Autodesk Inventor part; units mm, degrees
(part 3 of 3)
sketch "Эскиз4" plane through (0, 0, 0) normal (0, 0, -1) x (-1, 0, 0)
  arc A0 (-8.5879, 10.673) -> (-10.7903, 9.2375) centre (-9.1909, 9.1909) ccw
  line L0 (-8.8865, 7.6202) -> (-10.7903, 9.2375)
  arc A1 (-8.8865, 7.6202) -> (-7.8258, 10.0255) centre (-9.1909, 9.1909) ccw
  line L1 (-7.2868, 10.66) -> (-7.8258, 10.0255)
  line L2 (-8.5879, 10.673) -> (-8.0489, 11.3074)
  line L3 (-8.185, 11.3816) -> (-8.0489, 11.3074)
  line L4 (-8.4933, 11.4983) -> (-8.185, 11.3816)
  line L5 (-9.1961, 12.0463) -> (-8.4933, 11.4983)
  line L6 (-9.9839, 14.2526) -> (-9.1961, 12.0463)
  line L7 (-9.6596, 14.7646) -> (-9.9839, 14.2526)
  line L8 (-9.2928, 14.7834) -> (-9.6596, 14.7646)
  line L9 (-8.9255, 14.778) -> (-9.2928, 14.7834)
  line L10 (-8.5594, 14.7485) -> (-8.9255, 14.778)
  line L11 (-8.196, 14.6951) -> (-8.5594, 14.7485)
  line L12 (-7.837, 14.618) -> (-8.196, 14.6951)
  line L13 (-7.4837, 14.5174) -> (-7.837, 14.618)
  line L14 (-7.1378, 14.3939) -> (-7.4837, 14.5174)
  line L15 (-6.8007, 14.2479) -> (-7.1378, 14.3939)
  line L16 (-6.474, 14.0801) -> (-6.8007, 14.2479)
  line L17 (-6.159, 13.8913) -> (-6.474, 14.0801)
  line L18 (-5.857, 13.6822) -> (-6.159, 13.8913)
  line L19 (-5.5695, 13.4537) -> (-5.857, 13.6822)
  line L20 (-5.2975, 13.2068) -> (-5.5695, 13.4537)
  line L21 (-5.0423, 12.9426) -> (-5.2975, 13.2068)
  line L22 (-4.8051, 12.6623) -> (-5.0423, 12.9426)
  line L23 (-4.5867, 12.3669) -> (-4.8051, 12.6623)
  line L24 (-4.3882, 12.0579) -> (-4.5867, 12.3669)
  line L25 (-4.2104, 11.7365) -> (-4.3882, 12.0579)
  line L26 (-4.0541, 11.4041) -> (-4.2104, 11.7365)
  line L27 (-3.9199, 11.0622) -> (-4.0541, 11.4041)
  line L28 (-3.8084, 10.7123) -> (-3.9199, 11.0622)
  line L29 (-3.7202, 10.3557) -> (-3.8084, 10.7123)
  line L30 (-3.6555, 9.9942) -> (-3.7202, 10.3557)
  line L31 (-3.6147, 9.6291) -> (-3.6555, 9.9942)
  line L32 (-4.0677, 9.2263) -> (-3.6147, 9.6291)
  line L33 (-6.3723, 9.6472) -> (-4.0677, 9.2263)
  line L34 (-7.0266, 10.2523) -> (-6.3723, 9.6472)
  line L35 (-7.1917, 10.5377) -> (-7.0266, 10.2523)
  line L36 (-7.2868, 10.66) -> (-7.1917, 10.5377)
  line L37 (-7.2868, 10.66) -> (-7.8258, 10.0255)
  arc A2 (-8.8865, 7.6202) -> (-7.8258, 10.0255) centre (-9.1909, 9.1909) ccw
  line L38 (-8.8865, 7.6202) -> (-10.7903, 9.2375)
  arc A3 (-8.5879, 10.673) -> (-10.7903, 9.2375) centre (-9.1909, 9.1909) ccw
  line L39 (-8.5848, 2.046) -> (-8.6119, 2.08)
  line L40 (-8.5619, 2.0118) -> (-8.5848, 2.046)
  line L41 (-8.5252, 1.9426) -> (-8.5619, 2.0118)
  line L42 (-8.4969, 1.8728) -> (-8.5252, 1.9426)
  line L43 (-8.4749, 1.8024) -> (-8.4969, 1.8728)
  line L44 (-8.4578, 1.7316) -> (-8.4749, 1.8024)
  line L45 (-8.4351, 1.5888) -> (-8.4578, 1.7316)
  line L46 (-8.3988, 1.4474) -> (-8.4351, 1.5888)
  line L47 (-8.348, 1.3076) -> (-8.3988, 1.4474)
  line L48 (-8.2864, 1.1692) -> (-8.348, 1.3076)
  line L49 (-8.2156, 1.0322) -> (-8.2864, 1.1692)
  line L50 (-8.1367, 0.8965) -> (-8.2156, 1.0322)
  line L51 (-8.0501, 0.7623) -> (-8.1367, 0.8965)
  line L52 (-7.9562, 0.6297) -> (-8.0501, 0.7623)
  line L53 (-7.8555, 0.4989) -> (-7.9562, 0.6297)
  line L54 (-7.7481, 0.3698) -> (-7.8555, 0.4989)
  line L55 (-7.6343, 0.2426) -> (-7.7481, 0.3698)
  line L56 (-7.5448, 0.1486) -> (-7.6343, 0.2426)
  line L57 (-6.9702, 0.2723) -> (-7.5448, 0.1486)
  line L58 (-6.9273, 0.3948) -> (-6.9702, 0.2723)
  line L59 (-6.8759, 0.5575) -> (-6.9273, 0.3948)
  line L60 (-6.8312, 0.7194) -> (-6.8759, 0.5575)
  line L61 (-6.7932, 0.8801) -> (-6.8312, 0.7194)
  line L62 (-6.7622, 1.0396) -> (-6.7932, 0.8801)
  line L63 (-6.7385, 1.1975) -> (-6.7622, 1.0396)
  line L64 (-6.7224, 1.3537) -> (-6.7385, 1.1975)
  line L65 (-6.7143, 1.5077) -> (-6.7224, 1.3537)
  line L66 (-6.7151, 1.6592) -> (-6.7143, 1.5077)
  line L67 (-6.7263, 1.8075) -> (-6.7151, 1.6592)
  line L68 (-6.7515, 1.9513) -> (-6.7263, 1.8075)
  line L69 (-6.7895, 2.0908) -> (-6.7515, 1.9513)
  line L70 (-6.8031, 2.1623) -> (-6.7895, 2.0908)
  line L71 (-6.812, 2.2355) -> (-6.8031, 2.1623)
  line L72 (-6.8149, 2.3108) -> (-6.812, 2.2355)
  line L73 (-6.8099, 2.389) -> (-6.8149, 2.3108)
  line L74 (-6.8032, 2.4296) -> (-6.8099, 2.389)
  line L75 (-6.7924, 2.4717) -> (-6.8032, 2.4296)
  line L76 (-6.7757, 2.516) -> (-6.7924, 2.4717)
  line L77 (-6.7479, 2.5646) -> (-6.7757, 2.516)
  line L78 (-6.6571, 2.6374) -> (-6.7479, 2.5646)
  line L79 (-6.1482, 2.8577) -> (-6.6571, 2.6374)
  line L80 (-6.0329, 2.874) -> (-6.1482, 2.8577)
  line L81 (-5.9785, 2.861) -> (-6.0329, 2.874)
  line L82 (-5.9347, 2.8428) -> (-5.9785, 2.861)
  line L83 (-5.8967, 2.8219) -> (-5.9347, 2.8428)
  line L84 (-5.8625, 2.799) -> (-5.8967, 2.8219)
  line L85 (-5.8021, 2.7491) -> (-5.8625, 2.799)
  line L86 (-5.7492, 2.6954) -> (-5.8021, 2.7491)
  line L87 (-5.7019, 2.6389) -> (-5.7492, 2.6954)
  line L88 (-5.6591, 2.5799) -> (-5.7019, 2.6389)
  line L89 (-5.5834, 2.4568) -> (-5.6591, 2.5799)
  line L90 (-5.4958, 2.34) -> (-5.5834, 2.4568)
  line L91 (-5.3953, 2.2303) -> (-5.4958, 2.34)
  line L92 (-5.2855, 2.126) -> (-5.3953, 2.2303)
  line L93 (-5.1677, 2.0265) -> (-5.2855, 2.126)
  line L94 (-5.0428, 1.9313) -> (-5.1677, 2.0265)
  line L95 (-4.9114, 1.8405) -> (-5.0428, 1.9313)
  line L96 (-4.774, 1.7539) -> (-4.9114, 1.8405)
  line L97 (-4.6308, 1.6716) -> (-4.774, 1.7539)
  line L98 (-4.4822, 1.5934) -> (-4.6308, 1.6716)
  line L99 (-4.3284, 1.5195) -> (-4.4822, 1.5934)
  line L100 (-4.2097, 1.4669) -> (-4.3284, 1.5195)
  line L101 (-3.7262, 1.8011) -> (-4.2097, 1.4669)
  line L102 (-3.7335, 1.9306) -> (-3.7262, 1.8011)
  line L103 (-3.7483, 2.1006) -> (-3.7335, 1.9306)
  line L104 (-3.7689, 2.2673) -> (-3.7483, 2.1006)
  line L105 (-3.7953, 2.4303) -> (-3.7689, 2.2673)
  line L106 (-3.8277, 2.5895) -> (-3.7953, 2.4303)
  line L107 (-3.8662, 2.7445) -> (-3.8277, 2.5895)
  line L108 (-3.9111, 2.8949) -> (-3.8662, 2.7445)
  line L109 (-3.9626, 3.0403) -> (-3.9111, 2.8949)
  line L110 (-4.0213, 3.18) -> (-3.9626, 3.0403)
  line L111 (-4.0884, 3.3127) -> (-4.0213, 3.18)
  line L112 (-4.1667, 3.4359) -> (-4.0884, 3.3127)
  line L113 (-4.2551, 3.5502) -> (-4.1667, 3.4359)
  line L114 (-4.2951, 3.6112) -> (-4.2551, 3.5502)
  line L115 (-4.3313, 3.6754) -> (-4.2951, 3.6112)
  line L116 (-4.3629, 3.7438) -> (-4.3313, 3.6754)
  line L117 (-4.3881, 3.8179) -> (-4.3629, 3.7438)
  line L118 (-4.3975, 3.858) -> (-4.3881, 3.8179)
  line L119 (-4.4036, 3.901) -> (-4.3975, 3.858)
  line L120 (-4.4051, 3.9484) -> (-4.4036, 3.901)
  line L121 (-4.398, 4.0039) -> (-4.4051, 3.9484)
  line L122 (-4.3421, 4.106) -> (-4.398, 4.0039)
  line L123 (-3.9562, 4.5042) -> (-4.3421, 4.106)
  line L124 (-3.8559, 4.5633) -> (-3.9562, 4.5042)
  line L125 (-3.8007, 4.5722) -> (-3.8559, 4.5633)
  line L126 (-3.7533, 4.5722) -> (-3.8007, 4.5722)
  line L127 (-3.7101, 4.5673) -> (-3.7533, 4.5722)
  line L128 (-3.6697, 4.5593) -> (-3.7101, 4.5673)
  line L129 (-3.5949, 4.5364) -> (-3.6697, 4.5593)
  line L130 (-3.5255, 4.507) -> (-3.5949, 4.5364)
  line L131 (-3.4601, 4.4728) -> (-3.5255, 4.507)
  line L132 (-3.398, 4.4348) -> (-3.4601, 4.4728)
  line L133 (-3.2809, 4.3499) -> (-3.398, 4.4348)
  line L134 (-3.1554, 4.2755) -> (-3.2809, 4.3499)
  line L135 (-3.0205, 4.2127) -> (-3.1554, 4.2755)
  line L136 (-2.8791, 4.1584) -> (-3.0205, 4.2127)
  line L137 (-2.7322, 4.1115) -> (-2.8791, 4.1584)
  line L138 (-2.5804, 4.0714) -> (-2.7322, 4.1115)
  line L139 (-2.4243, 4.0377) -> (-2.5804, 4.0714)
  line L140 (-2.2642, 4.0103) -> (-2.4243, 4.0377)
  line L141 (-2.1004, 3.989) -> (-2.2642, 4.0103)
  line L142 (-1.9332, 3.9737) -> (-2.1004, 3.989)
  line L143 (-1.7628, 3.9643) -> (-1.9332, 3.9737)
  line L144 (-1.6331, 3.961) -> (-1.7628, 3.9643)
  line L145 (-1.3142, 4.4548) -> (-1.6331, 3.961)
  line L146 (-1.3705, 4.5717) -> (-1.3142, 4.4548)
  line L147 (-1.4492, 4.7232) -> (-1.3705, 4.5717)
  line L148 (-1.532, 4.8692) -> (-1.4492, 4.7232)
  line L149 (-1.6189, 5.0098) -> (-1.532, 4.8692)
  line L150 (-1.7097, 5.1444) -> (-1.6189, 5.0098)
  line L151 (-1.8046, 5.2729) -> (-1.7097, 5.1444)
  line L152 (-1.9036, 5.3947) -> (-1.8046, 5.2729)
  line L153 (-2.0068, 5.5093) -> (-1.9036, 5.3947)
  line L154 (-2.1145, 5.6158) -> (-2.0068, 5.5093)
  line L155 (-2.2273, 5.7129) -> (-2.1145, 5.6158)
  line L156 (-2.3468, 5.7967) -> (-2.2273, 5.7129)
  line L157 (-2.4723, 5.8685) -> (-2.3468, 5.7967)
  line L158 (-2.5325, 5.9094) -> (-2.4723, 5.8685)
  line L159 (-2.5905, 5.9549) -> (-2.5325, 5.9094)
  line L160 (-2.6459, 6.0061) -> (-2.5905, 5.9549)
  line L161 (-2.6976, 6.0649) -> (-2.6459, 6.0061)
  line L162 (-2.7215, 6.0983) -> (-2.6976, 6.0649)
  line L163 (-2.7437, 6.1357) -> (-2.7215, 6.0983)
  line L164 (-2.7632, 6.1789) -> (-2.7437, 6.1357)
  line L165 (-2.7779, 6.2329) -> (-2.7632, 6.1789)
  line L166 (-2.7652, 6.3486) -> (-2.7779, 6.2329)
  line L167 (-2.5611, 6.8642) -> (-2.7652, 6.3486)
  line L168 (-2.4911, 6.9572) -> (-2.5611, 6.8642)
  line L169 (-2.4434, 6.9865) -> (-2.4911, 6.9572)
  line L170 (-2.3996, 7.0047) -> (-2.4434, 6.9865)
  line L171 (-2.3579, 7.0167) -> (-2.3996, 7.0047)
  line L172 (-2.3175, 7.0247) -> (-2.3579, 7.0167)
  line L173 (-2.2396, 7.0322) -> (-2.3175, 7.0247)
  line L174 (-2.1643, 7.0316) -> (-2.2396, 7.0322)
  line L175 (-2.0908, 7.025) -> (-2.1643, 7.0316)
  line L176 (-2.0188, 7.0137) -> (-2.0908, 7.025)
  line L177 (-1.8782, 6.9801) -> (-2.0188, 7.0137)
  line L178 (-1.7338, 6.9594) -> (-1.8782, 6.9801)
  line L179 (-1.5851, 6.9529) -> (-1.7338, 6.9594)
  line L180 (-1.4337, 6.9569) -> (-1.5851, 6.9529)
  line L181 (-1.28, 6.9698) -> (-1.4337, 6.9569)
  line L182 (-1.1244, 6.9908) -> (-1.28, 6.9698)
  line L183 (-0.9673, 7.0195) -> (-1.1244, 6.9908)
  line L184 (-0.8089, 7.0554) -> (-0.9673, 7.0195)
  line L185 (-0.6494, 7.0984) -> (-0.8089, 7.0554)
  line L186 (-0.4891, 7.1482) -> (-0.6494, 7.0984)
  line L187 (-0.3281, 7.2047) -> (-0.4891, 7.1482)
  line L188 (-0.207, 7.2514) -> (-0.3281, 7.2047)
  line L189 (-0.1014, 7.8296) -> (-0.207, 7.2514)
  line L190 (-0.1981, 7.9161) -> (-0.1014, 7.8296)
  line L191 (-0.3288, 8.0259) -> (-0.1981, 7.9161)
  line L192 (-0.4612, 8.1291) -> (-0.3288, 8.0259)
  line L193 (-0.5952, 8.2257) -> (-0.4612, 8.1291)
  line L194 (-0.7307, 8.3154) -> (-0.5952, 8.2257)
  line L195 (-0.8675, 8.3977) -> (-0.7307, 8.3154)
  line L196 (-1.0056, 8.4724) -> (-0.8675, 8.3977)
  line L197 (-1.1448, 8.5388) -> (-1.0056, 8.4724)
  line L198 (-1.2851, 8.596) -> (-1.1448, 8.5388)
  line L199 (-1.4264, 8.6425) -> (-1.2851, 8.596)
  line L200 (-1.5688, 8.6742) -> (-1.4264, 8.6425)
  line L201 (-1.7122, 8.6925) -> (-1.5688, 8.6742)
  line L202 (-1.7836, 8.7073) -> (-1.7122, 8.6925)
  line L203 (-1.8546, 8.7271) -> (-1.7836, 8.7073)
  line L204 (-1.9253, 8.7532) -> (-1.8546, 8.7271)
  line L205 (-1.9955, 8.7878) -> (-1.9253, 8.7532)
  line L206 (-2.0305, 8.8095) -> (-1.9955, 8.7878)
  line L207 (-2.0653, 8.8355) -> (-2.0305, 8.8095)
  line L208 (-2.0998, 8.868) -> (-2.0653, 8.8355)
  line L209 (-2.1341, 8.9122) -> (-2.0998, 8.868)
  line L210 (-2.1666, 9.024) -> (-2.1341, 8.9122)
  line L211 (-2.1753, 9.5784) -> (-2.1666, 9.024)
  line L212 (-2.1463, 9.6911) -> (-2.1753, 9.5784)
  line L213 (-2.1135, 9.7365) -> (-2.1463, 9.6911)
  line L214 (-2.08, 9.77) -> (-2.1135, 9.7365)
  line L215 (-2.046, 9.7971) -> (-2.08, 9.77)
  line L216 (-2.0118, 9.8199) -> (-2.046, 9.7971)
  line L217 (-1.9426, 9.8567) -> (-2.0118, 9.8199)
  line L218 (-1.8728, 9.885) -> (-1.9426, 9.8567)
  line L219 (-1.8024, 9.907) -> (-1.8728, 9.885)
  line L220 (-1.7316, 9.924) -> (-1.8024, 9.907)
  line L221 (-1.5888, 9.9468) -> (-1.7316, 9.924)
  line L222 (-1.4474, 9.983) -> (-1.5888, 9.9468)
  line L223 (-1.3076, 10.0339) -> (-1.4474, 9.983)
  line L224 (-1.1692, 10.0955) -> (-1.3076, 10.0339)
  line L225 (-1.0322, 10.1662) -> (-1.1692, 10.0955)
  line L226 (-0.8965, 10.2452) -> (-1.0322, 10.1662)
  line L227 (-0.7623, 10.3318) -> (-0.8965, 10.2452)
  line L228 (-0.6297, 10.4256) -> (-0.7623, 10.3318)
  line L229 (-0.4989, 10.5264) -> (-0.6297, 10.4256)
  line L230 (-0.3698, 10.6338) -> (-0.4989, 10.5264)
  line L231 (-0.2426, 10.7476) -> (-0.3698, 10.6338)
  line L232 (-0.1486, 10.8371) -> (-0.2426, 10.7476)
  line L233 (-0.2723, 11.4117) -> (-0.1486, 10.8371)
  line L234 (-0.3948, 11.4545) -> (-0.2723, 11.4117)
  line L235 (-0.5575, 11.506) -> (-0.3948, 11.4545)
  line L236 (-0.7194, 11.5507) -> (-0.5575, 11.506)
  line L237 (-0.8801, 11.5887) -> (-0.7194, 11.5507)
  line L238 (-1.0396, 11.6196) -> (-0.8801, 11.5887)
  line L239 (-1.1975, 11.6434) -> (-1.0396, 11.6196)
  line L240 (-1.3537, 11.6595) -> (-1.1975, 11.6434)
  line L241 (-1.5077, 11.6676) -> (-1.3537, 11.6595)
  line L242 (-1.6592, 11.6667) -> (-1.5077, 11.6676)
  line L243 (-1.8075, 11.6556) -> (-1.6592, 11.6667)
  line L244 (-1.9513, 11.6304) -> (-1.8075, 11.6556)
  line L245 (-2.0908, 11.5924) -> (-1.9513, 11.6304)
  line L246 (-2.1623, 11.5788) -> (-2.0908, 11.5924)
  line L247 (-2.2355, 11.5699) -> (-2.1623, 11.5788)
  line L248 (-2.3108, 11.567) -> (-2.2355, 11.5699)
  line L249 (-2.389, 11.572) -> (-2.3108, 11.567)
  line L250 (-2.4296, 11.5787) -> (-2.389, 11.572)
  line L251 (-2.4717, 11.5894) -> (-2.4296, 11.5787)
  line L252 (-2.516, 11.6062) -> (-2.4717, 11.5894)
  line L253 (-2.5646, 11.634) -> (-2.516, 11.6062)
  line L254 (-2.6374, 11.7248) -> (-2.5646, 11.634)
  line L255 (-2.8577, 12.2337) -> (-2.6374, 11.7248)
  line L256 (-2.874, 12.3489) -> (-2.8577, 12.2337)
  line L257 (-2.861, 12.4034) -> (-2.874, 12.3489)
  line L258 (-2.8428, 12.4472) -> (-2.861, 12.4034)
  line L259 (-2.8219, 12.4852) -> (-2.8428, 12.4472)
  line L260 (-2.799, 12.5194) -> (-2.8219, 12.4852)
  line L261 (-2.7491, 12.5798) -> (-2.799, 12.5194)
  line L262 (-2.6954, 12.6327) -> (-2.7491, 12.5798)
  line L263 (-2.6389, 12.6799) -> (-2.6954, 12.6327)
  line L264 (-2.5799, 12.7228) -> (-2.6389, 12.6799)
  line L265 (-2.4568, 12.7985) -> (-2.5799, 12.7228)
  line L266 (-2.34, 12.886) -> (-2.4568, 12.7985)
  line L267 (-2.2303, 12.9865) -> (-2.34, 12.886)
  line L268 (-2.126, 13.0964) -> (-2.2303, 12.9865)
  line L269 (-2.0265, 13.2142) -> (-2.126, 13.0964)
  line L270 (-1.9313, 13.3391) -> (-2.0265, 13.2142)
  line L271 (-1.8405, 13.4704) -> (-1.9313, 13.3391)
  line L272 (-1.7539, 13.6079) -> (-1.8405, 13.4704)
  line L273 (-1.6716, 13.7511) -> (-1.7539, 13.6079)
  line L274 (-1.5934, 13.8997) -> (-1.6716, 13.7511)
  line L275 (-1.5195, 14.0535) -> (-1.5934, 13.8997)
  line L276 (-1.4669, 14.1721) -> (-1.5195, 14.0535)
  line L277 (-1.8011, 14.6556) -> (-1.4669, 14.1721)
  line L278 (-1.9306, 14.6484) -> (-1.8011, 14.6556)
  line L279 (-2.1006, 14.6336) -> (-1.9306, 14.6484)
  line L280 (-2.2673, 14.613) -> (-2.1006, 14.6336)
  line L281 (-2.4303, 14.5866) -> (-2.2673, 14.613)
  line L282 (-2.5895, 14.5541) -> (-2.4303, 14.5866)
  line L283 (-2.7445, 14.5156) -> (-2.5895, 14.5541)
  line L284 (-2.8949, 14.4708) -> (-2.7445, 14.5156)
  line L285 (-3.0403, 14.4193) -> (-2.8949, 14.4708)
  line L286 (-3.18, 14.3605) -> (-3.0403, 14.4193)
  line L287 (-3.3127, 14.2935) -> (-3.18, 14.3605)
  line L288 (-3.4359, 14.2152) -> (-3.3127, 14.2935)
  line L289 (-3.5502, 14.1267) -> (-3.4359, 14.2152)
  line L290 (-3.6112, 14.0868) -> (-3.5502, 14.1267)
  line L291 (-3.6754, 14.0505) -> (-3.6112, 14.0868)
  line L292 (-3.7438, 14.019) -> (-3.6754, 14.0505)
  line L293 (-3.8179, 13.9938) -> (-3.7438, 14.019)
  line L294 (-3.858, 13.9844) -> (-3.8179, 13.9938)
  line L295 (-3.901, 13.9782) -> (-3.858, 13.9844)
  line L296 (-3.9484, 13.9767) -> (-3.901, 13.9782)
  line L297 (-4.0039, 13.9838) -> (-3.9484, 13.9767)
  line L298 (-4.106, 14.0398) -> (-4.0039, 13.9838)
  line L299 (-4.5042, 14.4257) -> (-4.106, 14.0398)
  line L300 (-4.5633, 14.5259) -> (-4.5042, 14.4257)
  line L301 (-4.5722, 14.5812) -> (-4.5633, 14.5259)
  line L302 (-4.5722, 14.6286) -> (-4.5722, 14.5812)
  line L303 (-4.5673, 14.6718) -> (-4.5722, 14.6286)
  line L304 (-4.5593, 14.7121) -> (-4.5673, 14.6718)
  line L305 (-4.5364, 14.787) -> (-4.5593, 14.7121)
  line L306 (-4.507, 14.8564) -> (-4.5364, 14.787)
  line L307 (-4.4728, 14.9217) -> (-4.507, 14.8564)
  line L308 (-4.4348, 14.9839) -> (-4.4728, 14.9217)
  line L309 (-4.3499, 15.1009) -> (-4.4348, 14.9839)
  line L310 (-4.2755, 15.2265) -> (-4.3499, 15.1009)
  line L311 (-4.2127, 15.3613) -> (-4.2755, 15.2265)
  line L312 (-4.1584, 15.5028) -> (-4.2127, 15.3613)
  line L313 (-4.1115, 15.6497) -> (-4.1584, 15.5028)
  line L314 (-4.0714, 15.8015) -> (-4.1115, 15.6497)
  line L315 (-4.0377, 15.9576) -> (-4.0714, 15.8015)
  line L316 (-4.0103, 16.1177) -> (-4.0377, 15.9576)
  line L317 (-3.989, 16.2815) -> (-4.0103, 16.1177)
  line L318 (-3.9737, 16.4487) -> (-3.989, 16.2815)
  line L319 (-3.9643, 16.6191) -> (-3.9737, 16.4487)
  line L320 (-3.961, 16.7488) -> (-3.9643, 16.6191)
  line L321 (-4.4548, 17.0676) -> (-3.961, 16.7488)
  line L322 (-4.5717, 17.0113) -> (-4.4548, 17.0676)
  line L323 (-4.7232, 16.9326) -> (-4.5717, 17.0113)
  line L324 (-4.8692, 16.8498) -> (-4.7232, 16.9326)
  line L325 (-5.0098, 16.763) -> (-4.8692, 16.8498)
  line L326 (-5.1444, 16.6721) -> (-5.0098, 16.763)
  line L327 (-5.2729, 16.5772) -> (-5.1444, 16.6721)
  line L328 (-5.3947, 16.4783) -> (-5.2729, 16.5772)
  line L329 (-5.5093, 16.375) -> (-5.3947, 16.4783)
  line L330 (-5.6158, 16.2673) -> (-5.5093, 16.375)
  line L331 (-5.7129, 16.1546) -> (-5.6158, 16.2673)
  line L332 (-5.7967, 16.0351) -> (-5.7129, 16.1546)
  line L333 (-5.8685, 15.9096) -> (-5.7967, 16.0351)
  line L334 (-5.9094, 15.8494) -> (-5.8685, 15.9096)
  line L335 (-5.9549, 15.7913) -> (-5.9094, 15.8494)
  line L336 (-6.0061, 15.736) -> (-5.9549, 15.7913)
  line L337 (-6.0649, 15.6843) -> (-6.0061, 15.736)
  line L338 (-6.0983, 15.6603) -> (-6.0649, 15.6843)
  line L339 (-6.1357, 15.6382) -> (-6.0983, 15.6603)
  line L340 (-6.1789, 15.6187) -> (-6.1357, 15.6382)
  line L341 (-6.2329, 15.604) -> (-6.1789, 15.6187)
  line L342 (-6.3486, 15.6166) -> (-6.2329, 15.604)
  line L343 (-6.8642, 15.8208) -> (-6.3486, 15.6166)
  line L344 (-6.9572, 15.8907) -> (-6.8642, 15.8208)
  line L345 (-6.9865, 15.9384) -> (-6.9572, 15.8907)
  line L346 (-7.0047, 15.9822) -> (-6.9865, 15.9384)
  line L347 (-7.0167, 16.0239) -> (-7.0047, 15.9822)
  line L348 (-7.0247, 16.0643) -> (-7.0167, 16.0239)
  line L349 (-7.0322, 16.1423) -> (-7.0247, 16.0643)
  line L350 (-7.0316, 16.2176) -> (-7.0322, 16.1423)
  line L351 (-7.025, 16.2911) -> (-7.0316, 16.2176)
  line L352 (-7.0137, 16.363) -> (-7.025, 16.2911)
  line L353 (-6.9801, 16.5036) -> (-7.0137, 16.363)
  line L354 (-6.9594, 16.6481) -> (-6.9801, 16.5036)
  line L355 (-6.9529, 16.7967) -> (-6.9594, 16.6481)
  line L356 (-6.9569, 16.9482) -> (-6.9529, 16.7967)
  line L357 (-6.9698, 17.1019) -> (-6.9569, 16.9482)
  line L358 (-6.9908, 17.2574) -> (-6.9698, 17.1019)
  line L359 (-7.0195, 17.4145) -> (-6.9908, 17.2574)
  line L360 (-7.0554, 17.5729) -> (-7.0195, 17.4145)
  line L361 (-7.0984, 17.7324) -> (-7.0554, 17.5729)
  line L362 (-7.1482, 17.8928) -> (-7.0984, 17.7324)
  line L363 (-7.2047, 18.0538) -> (-7.1482, 17.8928)
  line L364 (-7.2514, 18.1749) -> (-7.2047, 18.0538)
  line L365 (-7.8296, 18.2805) -> (-7.2514, 18.1749)
  line L366 (-7.9161, 18.1837) -> (-7.8296, 18.2805)
  line L367 (-8.0259, 18.0531) -> (-7.9161, 18.1837)
  line L368 (-8.1291, 17.9207) -> (-8.0259, 18.0531)
  line L369 (-8.2257, 17.7867) -> (-8.1291, 17.9207)
  line L370 (-8.3154, 17.6512) -> (-8.2257, 17.7867)
  line L371 (-8.3977, 17.5144) -> (-8.3154, 17.6512)
  line L372 (-8.4724, 17.3763) -> (-8.3977, 17.5144)
  line L373 (-8.5388, 17.2371) -> (-8.4724, 17.3763)
  line L374 (-8.596, 17.0968) -> (-8.5388, 17.2371)
  line L375 (-8.6425, 16.9555) -> (-8.596, 17.0968)
  line L376 (-8.6742, 16.813) -> (-8.6425, 16.9555)
  line L377 (-8.6925, 16.6696) -> (-8.6742, 16.813)
  line L378 (-8.7073, 16.5983) -> (-8.6925, 16.6696)
  line L379 (-8.7271, 16.5273) -> (-8.7073, 16.5983)
  line L380 (-8.7532, 16.4566) -> (-8.7271, 16.5273)
  line L381 (-8.7878, 16.3863) -> (-8.7532, 16.4566)
  line L382 (-8.8095, 16.3514) -> (-8.7878, 16.3863)
  line L383 (-8.8355, 16.3166) -> (-8.8095, 16.3514)
  line L384 (-8.868, 16.282) -> (-8.8355, 16.3166)
  line L385 (-8.9122, 16.2478) -> (-8.868, 16.282)
  line L386 (-9.024, 16.2152) -> (-8.9122, 16.2478)
  line L387 (-9.5784, 16.2065) -> (-9.024, 16.2152)
  line L388 (-9.6911, 16.2356) -> (-9.5784, 16.2065)
  line L389 (-9.7365, 16.2684) -> (-9.6911, 16.2356)
  line L390 (-9.77, 16.3019) -> (-9.7365, 16.2684)
  line L391 (-9.7971, 16.3359) -> (-9.77, 16.3019)
  line L392 (-9.8199, 16.3701) -> (-9.7971, 16.3359)
  line L393 (-9.8567, 16.4393) -> (-9.8199, 16.3701)
  line L394 (-9.885, 16.5091) -> (-9.8567, 16.4393)
  line L395 (-9.907, 16.5795) -> (-9.885, 16.5091)
  line L396 (-9.924, 16.6503) -> (-9.907, 16.5795)
  line L397 (-9.9468, 16.7931) -> (-9.924, 16.6503)
  line L398 (-9.983, 16.9344) -> (-9.9468, 16.7931)
  line L399 (-10.0339, 17.0742) -> (-9.983, 16.9344)
  line L400 (-10.0955, 17.2126) -> (-10.0339, 17.0742)
  line L401 (-10.1662, 17.3497) -> (-10.0955, 17.2126)
  line L402 (-10.2452, 17.4854) -> (-10.1662, 17.3497)
  line L403 (-10.3318, 17.6195) -> (-10.2452, 17.4854)
  line L404 (-10.4256, 17.7521) -> (-10.3318, 17.6195)
  line L405 (-10.5264, 17.883) -> (-10.4256, 17.7521)
  line L406 (-10.6338, 18.0121) -> (-10.5264, 17.883)
  line L407 (-10.7476, 18.1392) -> (-10.6338, 18.0121)
  line L408 (-10.8371, 18.2332) -> (-10.7476, 18.1392)
  line L409 (-11.4117, 18.1095) -> (-10.8371, 18.2332)
  line L410 (-11.4545, 17.987) -> (-11.4117, 18.1095)
  line L411 (-11.506, 17.8243) -> (-11.4545, 17.987)
  line L412 (-11.5507, 17.6625) -> (-11.506, 17.8243)
  line L413 (-11.5887, 17.5017) -> (-11.5507, 17.6625)
  line L414 (-11.6196, 17.3423) -> (-11.5887, 17.5017)
  line L415 (-11.6434, 17.1843) -> (-11.6196, 17.3423)
  line L416 (-11.6595, 17.0282) -> (-11.6434, 17.1843)
  line L417 (-11.6676, 16.8742) -> (-11.6595, 17.0282)
  line L418 (-11.6667, 16.7227) -> (-11.6676, 16.8742)
  line L419 (-11.6556, 16.5743) -> (-11.6667, 16.7227)
  line L420 (-11.6304, 16.4306) -> (-11.6556, 16.5743)
  line L421 (-11.5924, 16.2911) -> (-11.6304, 16.4306)
  line L422 (-11.5788, 16.2195) -> (-11.5924, 16.2911)
  line L423 (-11.5699, 16.1463) -> (-11.5788, 16.2195)
  line L424 (-11.567, 16.071) -> (-11.5699, 16.1463)
  line L425 (-11.572, 15.9929) -> (-11.567, 16.071)
  line L426 (-11.5787, 15.9523) -> (-11.572, 15.9929)
  line L427 (-11.5894, 15.9102) -> (-11.5787, 15.9523)
  line L428 (-11.6062, 15.8658) -> (-11.5894, 15.9102)
  line L429 (-11.634, 15.8173) -> (-11.6062, 15.8658)
  line L430 (-11.7248, 15.7444) -> (-11.634, 15.8173)
  line L431 (-12.2337, 15.5242) -> (-11.7248, 15.7444)
  line L432 (-12.3489, 15.5079) -> (-12.2337, 15.5242)
  line L433 (-12.4034, 15.5209) -> (-12.3489, 15.5079)
  line L434 (-12.4472, 15.539) -> (-12.4034, 15.5209)
  line L435 (-12.4852, 15.56) -> (-12.4472, 15.539)
  line L436 (-12.5194, 15.5829) -> (-12.4852, 15.56)
  line L437 (-12.5798, 15.6327) -> (-12.5194, 15.5829)
  line L438 (-12.6327, 15.6864) -> (-12.5798, 15.6327)
  line L439 (-12.6799, 15.743) -> (-12.6327, 15.6864)
  line L440 (-12.7228, 15.8019) -> (-12.6799, 15.743)
  line L441 (-12.7985, 15.9251) -> (-12.7228, 15.8019)
  line L442 (-12.886, 16.0419) -> (-12.7985, 15.9251)
  line L443 (-12.9865, 16.1515) -> (-12.886, 16.0419)
  line L444 (-13.0964, 16.2558) -> (-12.9865, 16.1515)
  line L445 (-13.2142, 16.3554) -> (-13.0964, 16.2558)
  line L446 (-13.3391, 16.4505) -> (-13.2142, 16.3554)
  line L447 (-13.4704, 16.5413) -> (-13.3391, 16.4505)
  line L448 (-13.6079, 16.6279) -> (-13.4704, 16.5413)
  line L449 (-13.7511, 16.7103) -> (-13.6079, 16.6279)
  line L450 (-13.8997, 16.7885) -> (-13.7511, 16.7103)
  line L451 (-14.0535, 16.8624) -> (-13.8997, 16.7885)
  line L452 (-14.1721, 16.915) -> (-14.0535, 16.8624)
  line L453 (-14.6556, 16.5808) -> (-14.1721, 16.915)
  line L454 (-14.6484, 16.4512) -> (-14.6556, 16.5808)
  line L455 (-14.6336, 16.2812) -> (-14.6484, 16.4512)
  line L456 (-14.613, 16.1146) -> (-14.6336, 16.2812)
  line L457 (-14.5866, 15.9515) -> (-14.613, 16.1146)
  line L458 (-14.5541, 15.7924) -> (-14.5866, 15.9515)
  line L459 (-14.5156, 15.6374) -> (-14.5541, 15.7924)
  line L460 (-14.4708, 15.4869) -> (-14.5156, 15.6374)
  line L461 (-14.4193, 15.3416) -> (-14.4708, 15.4869)
  line L462 (-14.3605, 15.2019) -> (-14.4193, 15.3416)
  line L463 (-14.2935, 15.0691) -> (-14.3605, 15.2019)
  line L464 (-14.2152, 14.946) -> (-14.2935, 15.0691)
  line L465 (-14.1267, 14.8316) -> (-14.2152, 14.946)
  line L466 (-14.0868, 14.7707) -> (-14.1267, 14.8316)
  line L467 (-14.0505, 14.7065) -> (-14.0868, 14.7707)
  line L468 (-14.019, 14.638) -> (-14.0505, 14.7065)
  line L469 (-13.9938, 14.5639) -> (-14.019, 14.638)
  line L470 (-13.9844, 14.5238) -> (-13.9938, 14.5639)
  line L471 (-13.9782, 14.4809) -> (-13.9844, 14.5238)
  line L472 (-13.9767, 14.4335) -> (-13.9782, 14.4809)
  line L473 (-13.9838, 14.378) -> (-13.9767, 14.4335)
  line L474 (-14.0398, 14.2759) -> (-13.9838, 14.378)
  line L475 (-14.4257, 13.8777) -> (-14.0398, 14.2759)
  line L476 (-14.5259, 13.8185) -> (-14.4257, 13.8777)
  line L477 (-14.5812, 13.8097) -> (-14.5259, 13.8185)
  line L478 (-14.6286, 13.8097) -> (-14.5812, 13.8097)
  line L479 (-14.6718, 13.8145) -> (-14.6286, 13.8097)
  line L480 (-14.7121, 13.8226) -> (-14.6718, 13.8145)
  line L481 (-14.787, 13.8455) -> (-14.7121, 13.8226)
  line L482 (-14.8564, 13.8749) -> (-14.787, 13.8455)
  line L483 (-14.9217, 13.9091) -> (-14.8564, 13.8749)
  line L484 (-14.9839, 13.9471) -> (-14.9217, 13.9091)
  line L485 (-15.1009, 14.032) -> (-14.9839, 13.9471)
  line L486 (-15.2265, 14.1063) -> (-15.1009, 14.032)
  line L487 (-15.3613, 14.1692) -> (-15.2265, 14.1063)
  line L488 (-15.5028, 14.2235) -> (-15.3613, 14.1692)
  line L489 (-15.6497, 14.2704) -> (-15.5028, 14.2235)
  line L490 (-15.8015, 14.3105) -> (-15.6497, 14.2704)
  line L491 (-15.9576, 14.3441) -> (-15.8015, 14.3105)
  line L492 (-16.1177, 14.3715) -> (-15.9576, 14.3441)
  line L493 (-16.2815, 14.3928) -> (-16.1177, 14.3715)
  line L494 (-16.4487, 14.4082) -> (-16.2815, 14.3928)
  line L495 (-16.6191, 14.4176) -> (-16.4487, 14.4082)
  line L496 (-16.7488, 14.4208) -> (-16.6191, 14.4176)
  line L497 (-17.0676, 13.927) -> (-16.7488, 14.4208)
  line L498 (-17.0113, 13.8101) -> (-17.0676, 13.927)
  line L499 (-16.9326, 13.6587) -> (-17.0113, 13.8101)
  line L500 (-16.8498, 13.5126) -> (-16.9326, 13.6587)
  line L501 (-16.763, 13.3721) -> (-16.8498, 13.5126)
  line L502 (-16.6721, 13.2375) -> (-16.763, 13.3721)
  line L503 (-16.5772, 13.109) -> (-16.6721, 13.2375)
  line L504 (-16.4783, 12.9872) -> (-16.5772, 13.109)
  line L505 (-16.375, 12.8726) -> (-16.4783, 12.9872)
  line L506 (-16.2673, 12.766) -> (-16.375, 12.8726)
  line L507 (-16.1546, 12.669) -> (-16.2673, 12.766)
  line L508 (-16.0351, 12.5852) -> (-16.1546, 12.669)
  line L509 (-15.9096, 12.5134) -> (-16.0351, 12.5852)
  line L510 (-15.8494, 12.4724) -> (-15.9096, 12.5134)
  line L511 (-15.7913, 12.4269) -> (-15.8494, 12.4724)
  line L512 (-15.736, 12.3758) -> (-15.7913, 12.4269)
  line L513 (-15.6843, 12.317) -> (-15.736, 12.3758)
  line L514 (-15.6603, 12.2835) -> (-15.6843, 12.317)
  line L515 (-15.6382, 12.2462) -> (-15.6603, 12.2835)
  line L516 (-15.6187, 12.203) -> (-15.6382, 12.2462)
  line L517 (-15.604, 12.149) -> (-15.6187, 12.203)
  line L518 (-15.6166, 12.0333) -> (-15.604, 12.149)
  line L519 (-15.8208, 11.5177) -> (-15.6166, 12.0333)
  line L520 (-15.8907, 11.4247) -> (-15.8208, 11.5177)
  line L521 (-15.9384, 11.3953) -> (-15.8907, 11.4247)
  line L522 (-15.9822, 11.3772) -> (-15.9384, 11.3953)
  line L523 (-16.0239, 11.3651) -> (-15.9822, 11.3772)
  line L524 (-16.0643, 11.3572) -> (-16.0239, 11.3651)
  line L525 (-16.1423, 11.3497) -> (-16.0643, 11.3572)
  line L526 (-16.2176, 11.3503) -> (-16.1423, 11.3497)
  line L527 (-16.2911, 11.3568) -> (-16.2176, 11.3503)
  line L528 (-16.363, 11.3682) -> (-16.2911, 11.3568)
  line L529 (-16.5036, 11.4018) -> (-16.363, 11.3682)
  line L530 (-16.6481, 11.4224) -> (-16.5036, 11.4018)
  line L531 (-16.7967, 11.4289) -> (-16.6481, 11.4224)
  line L532 (-16.9482, 11.425) -> (-16.7967, 11.4289)
  line L533 (-17.1019, 11.4121) -> (-16.9482, 11.425)
  line L534 (-17.2574, 11.3911) -> (-17.1019, 11.4121)
  line L535 (-17.4145, 11.3624) -> (-17.2574, 11.3911)
  line L536 (-17.5729, 11.3264) -> (-17.4145, 11.3624)
  line L537 (-17.7324, 11.2834) -> (-17.5729, 11.3264)
  line L538 (-17.8928, 11.2336) -> (-17.7324, 11.2834)
  line L539 (-18.0538, 11.1771) -> (-17.8928, 11.2336)
  line L540 (-18.1749, 11.1304) -> (-18.0538, 11.1771)
  line L541 (-18.2805, 10.5522) -> (-18.1749, 11.1304)
  line L542 (-18.1837, 10.4658) -> (-18.2805, 10.5522)
  line L543 (-18.0531, 10.356) -> (-18.1837, 10.4658)
  line L544 (-17.9207, 10.2527) -> (-18.0531, 10.356)
  line L545 (-17.7867, 10.1561) -> (-17.9207, 10.2527)
  line L546 (-17.6512, 10.0665) -> (-17.7867, 10.1561)
  line L547 (-17.5144, 9.9841) -> (-17.6512, 10.0665)
  line L548 (-17.3763, 9.9095) -> (-17.5144, 9.9841)
  line L549 (-17.2371, 9.8431) -> (-17.3763, 9.9095)
  line L550 (-17.0968, 9.7859) -> (-17.2371, 9.8431)
  line L551 (-16.9555, 9.7394) -> (-17.0968, 9.7859)
  line L552 (-16.813, 9.7076) -> (-16.9555, 9.7394)
  line L553 (-16.6696, 9.6894) -> (-16.813, 9.7076)
  line L554 (-16.5983, 9.6746) -> (-16.6696, 9.6894)
  line L555 (-16.5273, 9.6547) -> (-16.5983, 9.6746)
  line L556 (-16.4566, 9.6287) -> (-16.5273, 9.6547)
  line L557 (-16.3863, 9.5941) -> (-16.4566, 9.6287)
  line L558 (-16.3514, 9.5724) -> (-16.3863, 9.5941)
  line L559 (-16.3166, 9.5464) -> (-16.3514, 9.5724)
  line L560 (-16.282, 9.5139) -> (-16.3166, 9.5464)
  line L561 (-16.2478, 9.4696) -> (-16.282, 9.5139)
  line L562 (-16.2152, 9.3579) -> (-16.2478, 9.4696)
  line L563 (-16.2065, 8.8034) -> (-16.2152, 9.3579)
  line L564 (-16.2356, 8.6907) -> (-16.2065, 8.8034)
  line L565 (-16.2684, 8.6454) -> (-16.2356, 8.6907)
  line L566 (-16.3019, 8.6119) -> (-16.2684, 8.6454)
  line L567 (-16.3359, 8.5848) -> (-16.3019, 8.6119)
  line L568 (-16.3701, 8.5619) -> (-16.3359, 8.5848)
  line L569 (-16.4393, 8.5252) -> (-16.3701, 8.5619)
  line L570 (-16.5091, 8.4969) -> (-16.4393, 8.5252)
  line L571 (-16.5795, 8.4749) -> (-16.5091, 8.4969)
  line L572 (-16.6503, 8.4578) -> (-16.5795, 8.4749)
  line L573 (-16.7931, 8.4351) -> (-16.6503, 8.4578)
  line L574 (-16.9344, 8.3988) -> (-16.7931, 8.4351)
  line L575 (-17.0742, 8.348) -> (-16.9344, 8.3988)
  line L576 (-17.2126, 8.2864) -> (-17.0742, 8.348)
  line L577 (-17.3497, 8.2156) -> (-17.2126, 8.2864)
  line L578 (-17.4854, 8.1367) -> (-17.3497, 8.2156)
  line L579 (-17.6195, 8.0501) -> (-17.4854, 8.1367)
  line L580 (-17.7521, 7.9562) -> (-17.6195, 8.0501)
  line L581 (-17.883, 7.8555) -> (-17.7521, 7.9562)
  line L582 (-18.0121, 7.7481) -> (-17.883, 7.8555)
  line L583 (-18.1392, 7.6343) -> (-18.0121, 7.7481)
  line L584 (-18.2332, 7.5448) -> (-18.1392, 7.6343)
  line L585 (-18.1095, 6.9702) -> (-18.2332, 7.5448)
  line L586 (-17.987, 6.9273) -> (-18.1095, 6.9702)
  line L587 (-17.8243, 6.8759) -> (-17.987, 6.9273)
  line L588 (-17.6625, 6.8312) -> (-17.8243, 6.8759)
  line L589 (-17.5017, 6.7932) -> (-17.6625, 6.8312)
  line L590 (-17.3423, 6.7622) -> (-17.5017, 6.7932)
  line L591 (-17.1843, 6.7385) -> (-17.3423, 6.7622)
  line L592 (-17.0282, 6.7224) -> (-17.1843, 6.7385)
  line L593 (-16.8742, 6.7143) -> (-17.0282, 6.7224)
  line L594 (-16.7227, 6.7151) -> (-16.8742, 6.7143)
  line L595 (-16.5743, 6.7263) -> (-16.7227, 6.7151)
  line L596 (-16.4306, 6.7515) -> (-16.5743, 6.7263)
  line L597 (-16.2911, 6.7895) -> (-16.4306, 6.7515)
  line L598 (-16.2195, 6.8031) -> (-16.2911, 6.7895)
  line L599 (-16.1463, 6.812) -> (-16.2195, 6.8031)
  line L600 (-16.071, 6.8149) -> (-16.1463, 6.812)
  line L601 (-15.9929, 6.8099) -> (-16.071, 6.8149)
  line L602 (-15.9523, 6.8032) -> (-15.9929, 6.8099)
  line L603 (-15.9102, 6.7924) -> (-15.9523, 6.8032)
  line L604 (-15.8658, 6.7757) -> (-15.9102, 6.7924)
  line L605 (-15.8173, 6.7479) -> (-15.8658, 6.7757)
  line L606 (-15.7444, 6.6571) -> (-15.8173, 6.7479)
  line L607 (-15.5242, 6.1482) -> (-15.7444, 6.6571)
  line L608 (-15.5079, 6.0329) -> (-15.5242, 6.1482)
  line L609 (-15.5209, 5.9785) -> (-15.5079, 6.0329)
  line L610 (-15.539, 5.9347) -> (-15.5209, 5.9785)
  line L611 (-15.56, 5.8967) -> (-15.539, 5.9347)
  line L612 (-15.5829, 5.8625) -> (-15.56, 5.8967)
  line L613 (-15.6327, 5.8021) -> (-15.5829, 5.8625)
  line L614 (-15.6864, 5.7492) -> (-15.6327, 5.8021)
  line L615 (-15.743, 5.7019) -> (-15.6864, 5.7492)
  line L616 (-15.8019, 5.6591) -> (-15.743, 5.7019)
  line L617 (-15.9251, 5.5834) -> (-15.8019, 5.6591)
  line L618 (-16.0419, 5.4958) -> (-15.9251, 5.5834)
  line L619 (-16.1515, 5.3953) -> (-16.0419, 5.4958)
  line L620 (-16.2558, 5.2855) -> (-16.1515, 5.3953)
  line L621 (-16.3554, 5.1677) -> (-16.2558, 5.2855)
  line L622 (-16.4505, 5.0428) -> (-16.3554, 5.1677)
  line L623 (-16.5413, 4.9114) -> (-16.4505, 5.0428)
  line L624 (-16.6279, 4.774) -> (-16.5413, 4.9114)
  line L625 (-16.7103, 4.6308) -> (-16.6279, 4.774)
  line L626 (-16.7885, 4.4822) -> (-16.7103, 4.6308)
  line L627 (-16.8624, 4.3284) -> (-16.7885, 4.4822)
  line L628 (-16.915, 4.2097) -> (-16.8624, 4.3284)
  line L629 (-16.5808, 3.7262) -> (-16.915, 4.2097)
  line L630 (-16.4512, 3.7335) -> (-16.5808, 3.7262)
  line L631 (-16.2812, 3.7483) -> (-16.4512, 3.7335)
  line L632 (-16.1146, 3.7689) -> (-16.2812, 3.7483)
  line L633 (-15.9515, 3.7953) -> (-16.1146, 3.7689)
  line L634 (-15.7924, 3.8277) -> (-15.9515, 3.7953)
  line L635 (-15.6374, 3.8662) -> (-15.7924, 3.8277)
  line L636 (-15.4869, 3.9111) -> (-15.6374, 3.8662)
  line L637 (-15.3416, 3.9626) -> (-15.4869, 3.9111)
  line L638 (-15.2019, 4.0213) -> (-15.3416, 3.9626)
  line L639 (-15.0691, 4.0884) -> (-15.2019, 4.0213)
  line L640 (-14.946, 4.1667) -> (-15.0691, 4.0884)
  line L641 (-14.8316, 4.2551) -> (-14.946, 4.1667)
  line L642 (-14.7707, 4.2951) -> (-14.8316, 4.2551)
  line L643 (-14.7065, 4.3313) -> (-14.7707, 4.2951)
  line L644 (-14.638, 4.3629) -> (-14.7065, 4.3313)
  line L645 (-14.5639, 4.3881) -> (-14.638, 4.3629)
  line L646 (-14.5238, 4.3975) -> (-14.5639, 4.3881)
  line L647 (-14.4809, 4.4036) -> (-14.5238, 4.3975)
  line L648 (-14.4335, 4.4051) -> (-14.4809, 4.4036)
  line L649 (-14.378, 4.398) -> (-14.4335, 4.4051)
  line L650 (-14.2759, 4.3421) -> (-14.378, 4.398)
  line L651 (-13.8777, 3.9562) -> (-14.2759, 4.3421)
  line L652 (-13.8185, 3.8559) -> (-13.8777, 3.9562)
  line L653 (-13.8097, 3.8007) -> (-13.8185, 3.8559)
  line L654 (-13.8097, 3.7533) -> (-13.8097, 3.8007)
  line L655 (-13.8145, 3.7101) -> (-13.8097, 3.7533)
  line L656 (-13.8226, 3.6697) -> (-13.8145, 3.7101)
  line L657 (-13.8455, 3.5949) -> (-13.8226, 3.6697)
  line L658 (-13.8749, 3.5255) -> (-13.8455, 3.5949)
  line L659 (-13.9091, 3.4601) -> (-13.8749, 3.5255)
  line L660 (-13.9471, 3.398) -> (-13.9091, 3.4601)
  line L661 (-14.032, 3.2809) -> (-13.9471, 3.398)
  line L662 (-14.1063, 3.1554) -> (-14.032, 3.2809)
  line L663 (-14.1692, 3.0205) -> (-14.1063, 3.1554)
  line L664 (-14.2235, 2.8791) -> (-14.1692, 3.0205)
  line L665 (-14.2704, 2.7322) -> (-14.2235, 2.8791)
  line L666 (-14.3105, 2.5804) -> (-14.2704, 2.7322)
  line L667 (-14.3441, 2.4243) -> (-14.3105, 2.5804)
  line L668 (-14.3715, 2.2642) -> (-14.3441, 2.4243)
  line L669 (-14.3928, 2.1004) -> (-14.3715, 2.2642)
  line L670 (-14.4082, 1.9332) -> (-14.3928, 2.1004)
  line L671 (-14.4176, 1.7628) -> (-14.4082, 1.9332)
  line L672 (-14.4208, 1.6331) -> (-14.4176, 1.7628)
  line L673 (-13.927, 1.3142) -> (-14.4208, 1.6331)
  line L674 (-13.8101, 1.3705) -> (-13.927, 1.3142)
  line L675 (-13.6587, 1.4492) -> (-13.8101, 1.3705)
  line L676 (-13.5126, 1.532) -> (-13.6587, 1.4492)
  line L677 (-13.3721, 1.6189) -> (-13.5126, 1.532)
  line L678 (-13.2375, 1.7097) -> (-13.3721, 1.6189)
  line L679 (-13.109, 1.8046) -> (-13.2375, 1.7097)
  line L680 (-12.9872, 1.9036) -> (-13.109, 1.8046)
  line L681 (-12.8726, 2.0068) -> (-12.9872, 1.9036)
  line L682 (-12.766, 2.1145) -> (-12.8726, 2.0068)
  line L683 (-12.669, 2.2273) -> (-12.766, 2.1145)
  line L684 (-12.5852, 2.3468) -> (-12.669, 2.2273)
  line L685 (-12.5134, 2.4723) -> (-12.5852, 2.3468)
  line L686 (-12.4724, 2.5325) -> (-12.5134, 2.4723)
  line L687 (-12.4269, 2.5905) -> (-12.4724, 2.5325)
  line L688 (-12.3758, 2.6459) -> (-12.4269, 2.5905)
  line L689 (-12.317, 2.6976) -> (-12.3758, 2.6459)
  line L690 (-12.2835, 2.7215) -> (-12.317, 2.6976)
  line L691 (-12.2462, 2.7437) -> (-12.2835, 2.7215)
  line L692 (-12.203, 2.7632) -> (-12.2462, 2.7437)
  line L693 (-12.149, 2.7779) -> (-12.203, 2.7632)
  line L694 (-12.0333, 2.7652) -> (-12.149, 2.7779)
  line L695 (-11.5177, 2.5611) -> (-12.0333, 2.7652)
  line L696 (-11.4247, 2.4911) -> (-11.5177, 2.5611)
  line L697 (-11.3953, 2.4434) -> (-11.4247, 2.4911)
  line L698 (-11.3772, 2.3996) -> (-11.3953, 2.4434)
  line L699 (-11.3651, 2.3579) -> (-11.3772, 2.3996)
  line L700 (-11.3572, 2.3175) -> (-11.3651, 2.3579)
  line L701 (-11.3497, 2.2396) -> (-11.3572, 2.3175)
  line L702 (-11.3503, 2.1643) -> (-11.3497, 2.2396)
  line L703 (-11.3568, 2.0908) -> (-11.3503, 2.1643)
  line L704 (-11.3682, 2.0188) -> (-11.3568, 2.0908)
  line L705 (-11.4018, 1.8782) -> (-11.3682, 2.0188)
  line L706 (-11.4224, 1.7338) -> (-11.4018, 1.8782)
  line L707 (-11.4289, 1.5851) -> (-11.4224, 1.7338)
  line L708 (-11.425, 1.4337) -> (-11.4289, 1.5851)
  line L709 (-11.4121, 1.28) -> (-11.425, 1.4337)
  line L710 (-11.3911, 1.1244) -> (-11.4121, 1.28)
  line L711 (-11.3624, 0.9673) -> (-11.3911, 1.1244)
  line L712 (-11.3264, 0.8089) -> (-11.3624, 0.9673)
  line L713 (-11.2834, 0.6494) -> (-11.3264, 0.8089)
  line L714 (-11.2336, 0.4891) -> (-11.2834, 0.6494)
  line L715 (-11.1771, 0.3281) -> (-11.2336, 0.4891)
  line L716 (-11.1304, 0.207) -> (-11.1771, 0.3281)
  line L717 (-10.5522, 0.1014) -> (-11.1304, 0.207)
  line L718 (-10.4658, 0.1981) -> (-10.5522, 0.1014)
  line L719 (-10.356, 0.3288) -> (-10.4658, 0.1981)
  line L720 (-10.2527, 0.4612) -> (-10.356, 0.3288)
  line L721 (-10.1561, 0.5952) -> (-10.2527, 0.4612)
  line L722 (-10.0665, 0.7307) -> (-10.1561, 0.5952)
  line L723 (-9.9841, 0.8675) -> (-10.0665, 0.7307)
  line L724 (-9.9095, 1.0056) -> (-9.9841, 0.8675)
  line L725 (-9.8431, 1.1448) -> (-9.9095, 1.0056)
  line L726 (-9.7859, 1.2851) -> (-9.8431, 1.1448)
  line L727 (-9.7394, 1.4264) -> (-9.7859, 1.2851)
  line L728 (-9.7076, 1.5688) -> (-9.7394, 1.4264)
  line L729 (-9.6894, 1.7122) -> (-9.7076, 1.5688)
  line L730 (-9.6746, 1.7836) -> (-9.6894, 1.7122)
  line L731 (-9.6547, 1.8546) -> (-9.6746, 1.7836)
  line L732 (-9.6287, 1.9253) -> (-9.6547, 1.8546)
  line L733 (-9.5941, 1.9955) -> (-9.6287, 1.9253)
  line L734 (-9.5724, 2.0305) -> (-9.5941, 1.9955)
  line L735 (-9.5464, 2.0653) -> (-9.5724, 2.0305)
  line L736 (-9.5139, 2.0998) -> (-9.5464, 2.0653)
  line L737 (-9.4696, 2.1341) -> (-9.5139, 2.0998)
  line L738 (-9.3579, 2.1666) -> (-9.4696, 2.1341)
  line L739 (-8.8034, 2.1753) -> (-9.3579, 2.1666)
  line L740 (-8.6907, 2.1463) -> (-8.8034, 2.1753)
  line L741 (-8.6454, 2.1135) -> (-8.6907, 2.1463)
  line L742 (-8.6119, 2.08) -> (-8.6454, 2.1135)
  line L743 (-8.3803, 6.9208) -> (-8.6977, 6.8314)
  line L744 (-8.0781, 7.0526) -> (-8.3803, 6.9208)
  line L745 (-7.7968, 7.2245) -> (-8.0781, 7.0526)
  line L746 (-7.5415, 7.4331) -> (-7.7968, 7.2245)
  line L747 (-6.7155, 7.7678) -> (-7.5415, 7.4331)
  line L748 (-4.4109, 7.3469) -> (-6.7155, 7.7678)
  line L749 (-4.1296, 6.81) -> (-4.4109, 7.3469)
  line L750 (-4.2968, 6.4829) -> (-4.1296, 6.81)
  line L751 (-4.4851, 6.1676) -> (-4.2968, 6.4829)
  line L752 (-4.6936, 5.8652) -> (-4.4851, 6.1676)
  line L753 (-4.9216, 5.5772) -> (-4.6936, 5.8652)
  line L754 (-5.168, 5.3048) -> (-4.9216, 5.5772)
  line L755 (-5.4317, 5.0492) -> (-5.168, 5.3048)
  line L756 (-5.7116, 4.8114) -> (-5.4317, 5.0492)
  line L757 (-6.0066, 4.5925) -> (-5.7116, 4.8114)
  line L758 (-6.3152, 4.3934) -> (-6.0066, 4.5925)
  line L759 (-6.6363, 4.215) -> (-6.3152, 4.3934)
  line L760 (-6.9684, 4.0581) -> (-6.6363, 4.215)
  line L761 (-7.31, 3.9233) -> (-6.9684, 4.0581)
  line L762 (-7.6598, 3.8112) -> (-7.31, 3.9233)
  line L763 (-8.0162, 3.7223) -> (-7.6598, 3.8112)
  line L764 (-8.3776, 3.657) -> (-8.0162, 3.7223)
  line L765 (-8.7426, 3.6156) -> (-8.3776, 3.657)
  line L766 (-9.1094, 3.5981) -> (-8.7426, 3.6156)
  line L767 (-9.4767, 3.6049) -> (-9.1094, 3.5981)
  line L768 (-9.8427, 3.6357) -> (-9.4767, 3.6049)
  line L769 (-10.2059, 3.6904) -> (-9.8427, 3.6357)
  line L770 (-10.5647, 3.7689) -> (-10.2059, 3.6904)
  line L771 (-10.9176, 3.8707) -> (-10.5647, 3.7689)
  line L772 (-11.263, 3.9955) -> (-10.9176, 3.8707)
  line L773 (-11.5995, 4.1427) -> (-11.263, 3.9955)
  line L774 (-11.7219, 4.7363) -> (-11.5995, 4.1427)
  line L775 (-10.2051, 6.5218) -> (-11.7219, 4.7363)
  line L776 (-9.3539, 6.7859) -> (-10.2051, 6.5218)
  line L777 (-9.0243, 6.7862) -> (-9.3539, 6.7859)
  line L778 (-8.6977, 6.8314) -> (-9.0243, 6.7862)
  line L779 (-14.7474, 9.8325) -> (-14.7775, 9.4665)
  line L780 (-14.6933, 10.1958) -> (-14.7474, 9.8325)
  line L781 (-14.6155, 10.5548) -> (-14.6933, 10.1958)
  line L782 (-14.5143, 10.9079) -> (-14.6155, 10.5548)
  line L783 (-14.3901, 11.2535) -> (-14.5143, 10.9079)
  line L784 (-14.2435, 11.5903) -> (-14.3901, 11.2535)
  line L785 (-14.0752, 11.9168) -> (-14.2435, 11.5903)
  line L786 (-13.8857, 12.2314) -> (-14.0752, 11.9168)
  line L787 (-13.6761, 12.533) -> (-13.8857, 12.2314)
  line L788 (-13.4471, 12.8202) -> (-13.6761, 12.533)
  line L789 (-13.1997, 13.0917) -> (-13.4471, 12.8202)
  line L790 (-12.9351, 13.3463) -> (-13.1997, 13.0917)
  line L791 (-12.6543, 13.5831) -> (-12.9351, 13.3463)
  line L792 (-12.3585, 13.8009) -> (-12.6543, 13.5831)
  line L793 (-11.7832, 13.6101) -> (-12.3585, 13.8009)
  line L794 (-10.9954, 11.4038) -> (-11.7832, 13.6101)
  line L795 (-11.1922, 10.5346) -> (-10.9954, 11.4038)
  line L796 (-11.3569, 10.249) -> (-11.1922, 10.5346)
  line L797 (-11.481, 9.9435) -> (-11.3569, 10.249)
  line L798 (-11.5623, 9.624) -> (-11.481, 9.9435)
  line L799 (-11.5992, 9.2964) -> (-11.5623, 9.624)
  line L800 (-11.591, 8.9668) -> (-11.5992, 9.2964)
  line L801 (-11.538, 8.6414) -> (-11.591, 8.9668)
  line L802 (-11.6611, 7.7587) -> (-11.538, 8.6414)
  line L803 (-13.178, 5.9733) -> (-11.6611, 7.7587)
  line L804 (-13.7836, 5.9982) -> (-13.178, 5.9733)
  line L805 (-13.9832, 6.3065) -> (-13.7836, 5.9982)
  line L806 (-14.1622, 6.6272) -> (-13.9832, 6.3065)
  line L807 (-14.3197, 6.959) -> (-14.1622, 6.6272)
  line L808 (-14.4551, 7.3004) -> (-14.3197, 6.959)
  line L809 (-14.5679, 7.65) -> (-14.4551, 7.3004)
  line L810 (-14.6574, 8.0062) -> (-14.5679, 7.65)
  line L811 (-14.7234, 8.3675) -> (-14.6574, 8.0062)
  line L812 (-14.7655, 8.7324) -> (-14.7234, 8.3675)
  line L813 (-14.7836, 9.0993) -> (-14.7655, 8.7324)
  line L814 (-14.7775, 9.4665) -> (-14.7836, 9.0993)
  circle A4 centre (-9.1909, 9.1909) radius 2.8554
  point P0 (0, 0)
  point P1 (-11.6611, 7.7587)
  point P2 (-10.2051, 6.5218)
  point P3 (-6.3723, 9.6472)
  point P4 (-10.9954, 11.4038)
  constraints: 1 coincident, 3 other
extrude "Выдавливание4" add sketch "Эскиз4" along normal blind 4 contours A0 L0 A1 L1 L36 L35 L34 A4 L747 L746 L745 L744 L743 L778 L777 L776 L802 L801 L800 L799 L798 L797 L796 L795 L5 L4 L3 L2
